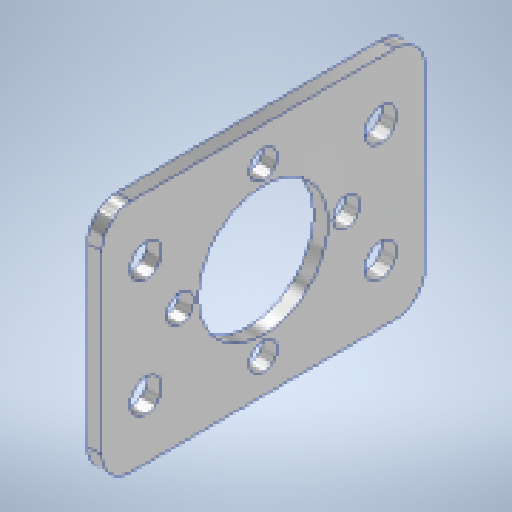
# Autodesk Inventor part: Motor Plates
Saved by Autodesk Inventor 2023.2 (Build 272271000, 271)
## iProperties
Created: 2022-05-26
Part Number: Motor Plates
Material: Aluminum 6061
Document SubType Name: Modeling
Designer: Nathan Cai
Density: 2.7 g/cm^3
Appearance: Aluminum - Flat
Mass: 3.74449 g
Surface Area: 21.5127 cm^2
Volume: 1.38685 cm^3
Author: Nathan Cai
Autodesk Inventor part; units mm, degrees
ref_plane "YZ Plane" through (0, 0, 0) normal (1, 0, 0) x (0, 1, 0)
ref_plane "XZ Plane" through (0, 0, 0) normal (0, 1, 0) x (-1, 0, 0)
ref_plane "XY Plane" through (0, 0, 0) normal (0, 0, 1) x (1, 0, 0)
sketch "Sketch1" plane through (0, 0, 0) normal (1, 0, 0) x (0, 1, 0)
  circle A0 centre (0, 0) radius 7
  line L0 (0, 0) -> (0, -12.7) construction
  line L1 (0, -12.7) -> (6.35, -12.7) construction
  circle A1 centre (6.35, -12.7) radius 1.7526
  circle A2 centre (-6.35, -12.7) radius 1.7526
  circle A3 centre (6.35, 12.7) radius 1.7526
  circle A4 centre (-6.35, 12.7) radius 1.7526
  line L2 (12.7, 17.4625) -> (-12.7, 17.4625)
  line L3 (-12.7, 17.4625) -> (-12.7, -17.4625)
  line L4 (-12.7, -17.4625) -> (12.7, -17.4625)
  line L5 (12.7, -17.4625) -> (12.7, 17.4625)
  line L6 (12.7, 17.4625) -> (-12.7, -17.4625) construction
  line L7 (-12.7, 17.4625) -> (12.7, -17.4625) construction
  circle A5 centre (9, 0) radius 1.5
  line L8 (0, 0) -> (9, 0) construction
  circle A6 centre (0, 9) radius 1.5
  circle A7 centre (-9, 0) radius 1.5
  circle A8 centre (0, -9) radius 1.5
  dimension "d0" = 14
  dimension "d1" = 12.7
  dimension "d2" = 6.35
  dimension "d3" = 3.5052
  dimension "d6" = 12.7
  dimension "d9" = 25.4
  dimension "d12" = 25.4
  dimension "d13" = 34.925
  dimension "d14" = 3
  dimension "d15" = 9
  dimension "d18" = 360
  constraints: 18 end point, 9 centre point, 4 horizontal, 3 midpoint, 2 coincident, 2 parallel, 2 vertical, 1 perpendicular, 15 other
  measures "d0" diameter of A0
  measures "d1" distance of L0.start L0.end
  measures "d2" distance of L0.end L1.end
  measures "d3" diameter of A1
  measures "d6" distance of A1.centre A2.centre
  measures "d9" distance of A1.centre A3.centre
  measures "d12" distance of L4.end L3.end
  measures "d13" distance of L3.end L2.end
  measures "d14" diameter of A5
  measures "d15" distance of L8.start L8.end
extrude "Extrusion1" add sketch "Sketch1" along normal blind 1.5875
fillet "Fillet1" radius 3.175 4 edges at (0.7937, 12.7, 17.4625) (0.7937, -12.7, 17.4625) (0.7937, 12.7, -17.4625) (0.7937, -12.7, -17.4625)
equation "\"d9\" = 2 * d1"
body "Solid1"
